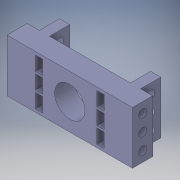
# Autodesk Inventor part: 000.404 - Переходник
Saved by Autodesk Inventor 2019 (Build 230136000, 136)
## iProperties
Created: 2020-02-28
Part Number: 000.404 - Переходник
Material: Пластик АБС
Document SubType Name: Modeling
Designer: Петров Иван
Density: 1.06 g/cm^3
Appearance: Грифельно-синий
Author: Петров Иван
Autodesk Inventor part; units mm, degrees
ref_plane "YZ Plane" through (0, 0, 0) normal (1, 0, 0) x (0, 1, 0)
ref_plane "XZ Plane" through (0, 0, 0) normal (0, 1, 0) x (-1, 0, 0)
ref_plane "XY Plane" through (0, 0, 0) normal (0, 0, 1) x (1, 0, 0)
sketch "Эскиз1" plane through (0, 0, 0) normal (0, 0, 1) x (1, 0, 0)
  line L0 (-30.974, -13.01) -> (30.974, -13.01)
  line L1 (30.974, -13.01) -> (30.974, 13.01)
  line L2 (30.974, 13.01) -> (-30.974, 13.01)
  line L3 (-30.974, 13.01) -> (-30.974, -13.01)
  line L4 (-30.974, -13.01) -> (30.974, 13.01) construction
  line L5 (30.974, -13.01) -> (-30.974, 13.01) construction
  point P0 (0, 0)
  dimension "d0" = 61.948
  dimension "d1" = 26.02
  constraints: 12 end point, 2 midpoint, 2 parallel, 1 horizontal, 1 perpendicular
  measures "d0" distance of L1.end L2.end
  measures "d1" distance of L0.end L1.end
extrude "Выдавливание1" add sketch "Эскиз1" along normal blind 10
sketch "Эскиз2" plane through (30.974, -13.01, 0) normal (1, 0, 0) x (0, 0, -1)
  line L0 (0, 13.01) -> (-5, 13.01)
  circle A0 centre (-5, 13.01) radius 2
  dimension "d4" = 5
  dimension "d5" = 4
  constraints: 2 end point, 1 centre point, 1 coincident, 1 horizontal
  measures "d4" distance of L0.start L0.end
  measures "d5" diameter of A0
extrude "Выдавливание2" cut sketch "Эскиз2" against normal blind 10
pattern_linear "Прямоуг.массив1" count 3 spacing 8 along (0, 1, 0) of "Выдавливание2" first direction both ways yes
mirror "Зеркальное отражение1" about plane through (0, 0, 0) normal (1, 0, 0) of "Выдавливание2", "Прямоуг.массив1"
sketch "Эскиз3" plane through (0, 0, 0) normal (0, 0, -1) x (-1, 0, 0)
  line L0 (0, 0) -> (-20, 0)
  line L1 (-30.974, 13.01) -> (30.974, 13.01) projected
  line L2 (30.974, -13.01) -> (-30.974, -13.01) projected
  line L3 (-20, 13.01) -> (-25, 13.01)
  line L4 (-25, 13.01) -> (-25, -13.01)
  line L5 (-25, -13.01) -> (-20, -13.01)
  line L6 (-20, -13.01) -> (-20, 13.01)
  line L7 (-30.974, -13.01) -> (-30.974, 13.01) projected
  dimension "d11" = 20
  dimension "d12" = 5
  constraints: 10 end point, 2 horizontal, 2 parallel, 2 point on line, 1 perpendicular
  measures "d11" distance of L0.start L0.end
  measures "d12" distance of L5.end L4.end
extrude "Выдавливание3" add sketch "Эскиз3" along normal blind 10 contours L1 L6 L2 L4
sketch "Эскиз4" plane through (25, -13.01, 0) normal (1, 0, 0) x (0, 0, -1)
  line L0 (10, 26.02) -> (10, 0) projected
  line L1 (10, 13.01) -> (5, 13.01)
  circle A0 centre (5, 13.01) radius 2
  point P0 (0, 13.01)
  dimension "d16" = 5
  dimension "d17" = 4
  constraints: 2 end point, 1 centre point, 1 coincident, 1 horizontal, 1 midpoint
  measures "d16" distance of L1.start L1.end
  measures "d17" diameter of A0
extrude "Выдавливание4" cut sketch "Эскиз4" against normal blind 10
pattern_linear "Прямоуг.массив2" count 3 spacing 8 along (0, -1, 0) of "Выдавливание4" first direction both ways yes
mirror "Зеркальное отражение2" about plane through (0, 0, 0) normal (1, 0, 0) of "Выдавливание3", "Выдавливание4", "Прямоуг.массив2"
sketch "Эскиз5" plane through (0, 0, 10) normal (0, 0, 1) x (1, 0, 0)
  circle A0 centre (0, 0) radius 7.5
  dimension "d23" = 15
  constraints: 1 centre point, 1 coincident
  measures "d23" diameter of A0
extrude "Выдавливание5" cut sketch "Эскиз5" against normal blind 23.75
sketch "Эскиз6" plane through (0, 0, 10) normal (0, 0, 1) x (1, 0, 0)
  circle A0 centre (0, 0) radius 5
  line L0 (-13.4261, 4.5029) -> (-16.9261, 4.5029)
  line L1 (-16.9261, 4.5029) -> (-16.9261, 11.4971)
  line L2 (-16.9261, 11.4971) -> (-13.4261, 11.4971)
  line L3 (-13.4261, 11.4971) -> (-13.4261, 4.5029)
  line L4 (-13.4261, -11.4971) -> (-16.9261, -11.4971)
  line L5 (-16.9261, -11.4971) -> (-16.9261, -4.5029)
  line L6 (-16.9261, -4.5029) -> (-13.4261, -4.5029)
  line L7 (-13.4261, -4.5029) -> (-13.4261, -11.4971)
  line L8 (-13.4261, -3.4971) -> (-16.9261, -3.4971)
  line L9 (-16.9261, -3.4971) -> (-16.9261, 3.4971)
  line L10 (-16.9261, 3.4971) -> (-13.4261, 3.4971)
  line L11 (-13.4261, 3.4971) -> (-13.4261, -3.4971)
  line L12 (10.5, 4.5029) -> (7, 4.5029)
  line L13 (7, 4.5029) -> (7, 11.4971)
  line L14 (7, 11.4971) -> (10.5, 11.4971)
  line L15 (10.5, 11.4971) -> (10.5, 4.5029)
  line L16 (10.5, -11.4971) -> (7, -11.4971)
  line L17 (7, -11.4971) -> (7, -4.5029)
  line L18 (7, -4.5029) -> (10.5, -4.5029)
  line L19 (10.5, -4.5029) -> (10.5, -11.4971)
  line L20 (7, 3.4971) -> (10.5, 3.4971)
  line L21 (10.5, 3.4971) -> (10.5, -3.4971)
  line L22 (10.5, -3.4971) -> (7, -3.4971)
  line L23 (7, -3.4971) -> (7, 3.4971)
  line L24 (17, -13.1) -> (17, 13.1)
  line L25 (17, 13.1) -> (-17, 13.1)
  line L26 (-17, 13.1) -> (-17, -13.1)
  line L27 (-17, -13.1) -> (17, -13.1)
  constraints: 56 end point, 1 centre point
extrude "Выдавливание6" cut sketch "Эскиз6" against normal blind 10 contours L0 L1 L2 L3 | L4 L5 L6 L7 | L8 L9 L10 L11
mirror "Зеркальное отражение3" about plane through (0, 0, 0) normal (1, 0, 0) of "Выдавливание6"
